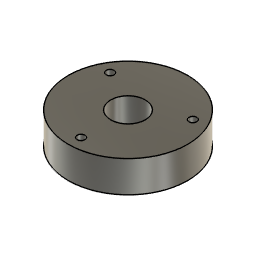
장민서 (Autodesk Fusion 360 design; units mm, degrees)
Autodesk Fusion 360 part; units mm, degrees
sketch "Sketch1" plane through (0, 0, 0) normal (0, 0, 1) x (1, 0, 0)
  circle A0 centre (0, 0) radius 11
  circle A1 centre (0, 0) radius 22.5
  circle A2 centre (0, 0) radius 38
  dimension "d1" = 45
  dimension "d2" = 22
  dimension "d3" = 76
  constraint coincident A0.centre A1.centre
  measures "d1" diameter of A1
  measures "d2" diameter of A0
  measures "d3" diameter of A2
extrude "Extrude1" add sketch "Sketch1" along normal blind 20 contours A1
sketch "Sketch2" plane through (0, 0, 0) normal (0, 0, 1) x (1, 0, 0)
  circle A0 centre (0.2654, -30.1553) radius 2.5
  dimension "d8" = 5
  measures "d8" diameter of A0
extrude "Extrude4" add sketch "Sketch1" along normal blind 2 contours A1 | A2
extrude "Extrude5" cut sketch "Sketch2" along normal blind 6.312
pattern_circular "C-Pattern2" count 3 over 360 about axis through (0, 0, 2) along (0, 0, 1) of "Extrude5"
extrude "돌출6" add 1 faces at (-20.8034, 21.3677, 2) along direction (0, 0, 1) blind 20
extrude "돌출7" cut 1 faces at (-20.8034, 21.3677, 22) along direction (0, 0, -1) blind 3
extrude "돌출8" add 1 faces at (-20.8034, 21.3677, 19) along direction (0, 0, 1) blind 1
